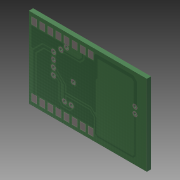
# Autodesk Inventor part: Bluetooth_module_PCB
Saved by Autodesk Inventor 2013 (Build 170138000, 138)
## iProperties
Created: 2015-07-02
Part Number: Bluetooth_module_PCB
Material: Ogólny
Document SubType Name: Modeling
Designer: terg
Density: 1 g/cm^3
Author: terg
Autodesk Inventor part; units mm, degrees
ref_plane "YZ Plane" through (0, 0, 0) normal (1, 0, 0) x (0, 1, 0)
ref_plane "XZ Plane" through (0, 0, 0) normal (0, 1, 0) x (-1, 0, 0)
ref_plane "XY Plane" through (0, 0, 0) normal (0, 0, 1) x (1, 0, 0)
sketch "Szkic1" plane through (0, 0, 0) normal (0, 1, 0) x (-1, 0, 0)
  line L0 (0, 0) -> (-22, 0)
  line L1 (-22, 0) -> (-22, -15)
  line L2 (-22, -15) -> (0, -15)
  line L3 (0, -15) -> (0, 0)
  dimension "d0" = 22
  dimension "d1" = 15
  constraints: 8 end point, 2 parallel, 1 horizontal, 1 perpendicular
  measures "d0" distance of L2.end L1.end
  measures "d1" distance of L1.end L0.end
extrude "Wyciągnięcie proste1" add sketch "Szkic1" along normal blind 0.8
sketch "Szkic2" plane through (0, 0.8, 0) normal (0, 1, 0) x (1, 0, 0)
  line L0 (0, 0) -> (22, 0) projected
  line L1 (22, 0) -> (22, 15) projected
  line L2 (22, 15) -> (0, 15) projected
  line L3 (0, 15) -> (0, 0) projected
  line L4 (-0.0247, 15) -> (22.0247, 15) construction
  line L5 (22.0247, 15) -> (22.0247, 0) construction
  line L6 (22.0247, 0) -> (-0.0247, 0) construction
  line L7 (-0.0247, 0) -> (-0.0247, 15) construction
  dimension "d9" = -0.0247
  dimension "d11" = 0
  dimension "d13" = 0
  dimension "d14" = -0.0247
  constraints: 2 other
  measures "d9" distance between parallel lines of L3 L7
  measures "d11" distance between parallel lines of L2 L4
  measures "d13" distance between parallel lines of L0 L6
  measures "d14" distance between parallel lines of L1 L5
decal "Pokrycie bitmapą1"
sketch "Szkic3" plane through (0, 0, 0) normal (0, -1, 0) x (1, 0, 0)
  line L0 (0, 0) -> (22, 0) projected
  line L1 (0, -15) -> (0, 0) projected
  line L2 (22, -15) -> (0, -15) projected
  line L3 (22, 0) -> (22, -15) projected
  line L4 (22.0408, -15) -> (-0.0408, -15) construction
  line L5 (-0.0408, -15) -> (-0.0408, 0) construction
  line L6 (-0.0408, 0) -> (22.0408, 0) construction
  line L7 (22.0408, 0) -> (22.0408, -15) construction
  dimension "d27" = -0.0408
  dimension "d28" = 0
  dimension "d31" = 0
  dimension "d32" = -0.0408
  constraints: 2 other
  measures "d27" distance between parallel lines of L3 L7
  measures "d28" distance between parallel lines of L2 L4
  measures "d31" distance between parallel lines of L0 L6
  measures "d32" distance between parallel lines of L1 L5
decal "Pokrycie bitmapą2"
sketch "Szkic5" plane through (0, 0.8, 0) normal (0, 1, 0) x (1, 0, 0)
  point P0 (4.635, 8.1423)
  point P1 (4.635, 6.8723)
  point P2 (4.635, 5.5876)
  point P3 (4.635, 4.3321)
  point P4 (6.0219, 3.3102)
  point P5 (7.0438, 2.4343)
  point P6 (8.3431, 7.3978)
  point P7 (6.6743, 11.3172)
  point P8 (7.959, 11.3172)
  point P9 (19.7924, 6.7985)
  point P10 (19.7924, 5.5876)
hole "Otwór2" at (4.635, 0.8, -8.1423) at (4.635, 0.8, -6.8723) at (4.635, 0.8, -5.5876) at (4.635, 0.8, -4.3321) at (6.0219, 0.8, -3.3102) at (7.0438, 0.8, -2.4343) at (8.3431, 0.8, -7.3978) at (6.6743, 0.8, -11.3172) at (7.959, 0.8, -11.3172) at (19.7924, 0.8, -6.7985) at (19.7924, 0.8, -5.5876) direction (0, -1, 0) diameter 0.4 depth 8
equation "\"d9\" = d14"
equation "\"d27\" = d32"
